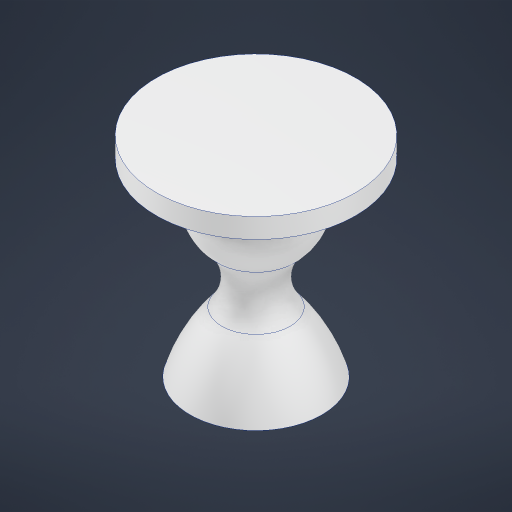
# Autodesk Inventor part: Liquid Engine
Saved by Autodesk Inventor 2023.2 (Build 272271030, 271C)
## iProperties
Created: 2023-04-10
Part Number: Liquid Engine
Material: Aluminum 6061
Document SubType Name: Modeling
Designer: ckeer
Density: 2.7 g/cm^3
Appearance: Aluminum - Flat
Author: ckeer
Autodesk Inventor part; units mm, degrees
ref_plane "YZ Plane" through (0, 0, 0) normal (1, 0, 0) x (0, 1, 0)
ref_plane "XZ Plane" through (0, 0, 0) normal (0, 1, 0) x (-1, 0, 0)
ref_plane "XY Plane" through (0, 0, 0) normal (0, 0, 1) x (1, 0, 0)
sketch "Sketch1" plane through (0, 0, 0) normal (0, 0, 1) x (1, 0, 0)
  line L0 (0, 0) -> (168.1535, 0)
  arc A0 (168.1535, 0) -> (86.9071, 154.7477) centre (-260.4145, -126.307) ccw
  arc A1 (96.2109, 298.6076) -> (86.9071, 154.7477) centre (169.5625, 221.6329) ccw
  arc A2 (96.2109, 298.6076) -> (127, 457.2) centre (0, 399.5708) ccw
  line L1 (127, 457.2) -> (0, 457.2)
  line L2 (0, 457.2) -> (0, 0)
  dimension "d0" = 457.2
  dimension "d1" = 127
  dimension "d2" = 0
  dimension "d3" = 0
  dimension "d5" = 446.793
  dimension "d6" = 106.3276
  dimension "d7" = 139.4637
  dimension "d8" = 169.5625
  dimension "d9" = 260.4145
  constraints: 6 end point, 6 point on circle, 3 centre point, 2 horizontal, 2 tangent
  measures "d0" distance of L0.start L1.end
  measures "d1" distance of L1.start L1.end
  measures "d2" horizontal distance of L0.start A2.centre
  measures "d3" horizontal distance of L0.start L1.end
  measures "d5" radius of A0
  measures "d6" radius of A1
  measures "d7" radius of A2
  measures "d8" distance from line of L2 A1.centre
  measures "d9" distance from line of L2 A0.centre
revolve "Revolution1" add sketch "Sketch1" angle 360 about axis through (0, 457.2, 0) along (0, -1, 0)
shell "Shell1" thickness 6.35 removed faces 1 at (-45.5245, 0, 42.2192)
sketch "Sketch2" plane through (0, 457.2, 0) normal (0, 1, 0) x (1, 0, 0)
  circle A0 centre (0, 0) radius 165.1
  dimension "d11" = 330.2
  constraints: 1 centre point, 1 coincident
  measures "d11" diameter of A0
extrude "Extrusion1" add sketch "Sketch2" along normal blind 25.4
sketch "Sketch3" plane through (0, 482.6, 0) normal (0, 1, 0) x (1, 0, 0)
  circle A0 centre (63.5, -63.5) radius 3.175
  point P0 (0, 0)
  dimension "d14" = 6.35
  dimension "d15" = 63.5
  dimension "d16" = 63.5
  constraints: 1 centre point
  measures "d14" diameter of A0
  measures "d15" horizontal distance of point (0, 0) A0.centre
  measures "d16" horizontal distance of A0.centre point (0, 0)
extrude "Extrusion2" cut sketch "Sketch3" against normal blind 25.4
pattern_circular "Circular Pattern1" count 20 over 360 about axis through (0, 221.6329, 0) along (0, -1, 0) of "Extrusion2"
sketch "Sketch4" plane through (0, 482.6, 0) normal (0, 1, 0) x (1, 0, 0)
  circle A0 centre (38.1, -38.1) radius 3.175
  point P0 (0, 0)
  dimension "d22" = 6.35
  dimension "d23" = 38.1
  dimension "d25" = 38.1
  constraints: 1 centre point
  measures "d22" diameter of A0
  measures "d23" horizontal distance of point (0, 0) A0.centre
  measures "d25" horizontal distance of point (0, 0) A0.centre
extrude "Extrusion3" cut sketch "Sketch4" against normal blind 25.4
pattern_circular "Circular Pattern2" count 15 over 360 about axis through (0, 221.6329, 0) along (0, -1, 0) of "Extrusion3"
sketch "Sketch5" plane through (0, 482.6, 0) normal (0, 1, 0) x (1, 0, 0)
  circle A0 centre (0, 0) radius 254
  dimension "d31" = 508
  constraints: 1 centre point, 1 coincident
  measures "d31" diameter of A0
extrude "Extrusion4" add sketch "Sketch5" along normal blind 50.8
body "Solid1"
